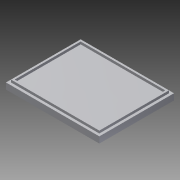
# Autodesk Inventor part: Pi Case Top V 01
Saved by Autodesk Inventor 2015 SP1 (Build 190203100, 203)
## iProperties
Created: 2015-03-22
Part Number: Pi Case Top V 01
Material: ABS Plastic
Document SubType Name: Modeling
Designer: steele
Density: 1.06 g/cm^3
Appearance: Smooth - White
Author: steele
Autodesk Inventor part; units mm, degrees
ref_plane "YZ Plane" through (0, 0, 0) normal (1, 0, 0) x (0, 1, 0)
ref_plane "XZ Plane" through (0, 0, 0) normal (0, 1, 0) x (-1, 0, 0)
ref_plane "XY Plane" through (0, 0, 0) normal (0, 0, 1) x (1, 0, 0)
sketch "Sketch1" plane through (0, 0, 0) normal (0, 0, 1) x (1, 0, 0)
  line L0 (-75, -60) -> (75, -60)
  line L1 (75, -60) -> (75, 60)
  line L2 (75, 60) -> (-75, 60)
  line L3 (-75, 60) -> (-75, -60)
  line L4 (-75, -60) -> (75, 60) construction
  line L5 (75, -60) -> (-75, 60) construction
  point P0 (0, 0)
  dimension "d0" = 150
  dimension "d1" = 120
  constraints: 12 end point, 2 midpoint, 2 parallel, 1 horizontal, 1 perpendicular
  measures "d0" distance of L0.start L0.end
  measures "d1" distance of L2.end L0.start
extrude "Extrusion1" add sketch "Sketch1" against normal blind 10
sketch "Sketch2" plane through (0, 0, 0) normal (0, 0, 1) x (1, 0, 0)
  line L0 (-71, -56) -> (71, -56)
  line L1 (71, -56) -> (71, 56)
  line L2 (71, 56) -> (-71, 56)
  line L3 (-71, 56) -> (-71, -56)
  line L4 (-71, -56) -> (71, 56) construction
  line L5 (71, -56) -> (-71, 56) construction
  line L6 (75, 60) -> (-75, 60) projected
  line L7 (-75, 60) -> (-75, -60) projected
  line L8 (-68, -53) -> (68, -53)
  line L9 (68, -53) -> (68, 53)
  line L10 (68, 53) -> (-68, 53)
  line L11 (-68, 53) -> (-68, -53)
  line L12 (-68, -53) -> (68, 53) construction
  line L13 (68, -53) -> (-68, 53) construction
  point P0 (0, 0)
  dimension "d4" = 4
  dimension "d5" = 4
  dimension "d6" = 3
  dimension "d7" = 3
  constraints: 24 end point, 4 midpoint, 4 parallel, 2 horizontal, 2 perpendicular
  measures "d4" distance between parallel lines of L2 L6
  measures "d5" distance between parallel lines of L3 L7
  measures "d6" distance between parallel lines of L2 L10
  measures "d7" distance between parallel lines of L3 L11
extrude "Extrusion2" add sketch "Sketch2" along normal blind 4
body "Solid1"
